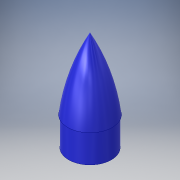
# Autodesk Inventor part: NoseCone
Saved by Autodesk Inventor 2018 (Build 220112000, 112)
## iProperties
Created: 2017-10-02
Part Number: NoseCone
Material: Generic
Document SubType Name: Modeling
Designer: Intel
Density: 1 g/cm^3
Appearance: Blue - Wall Paint - Glossy
Author: Intel
Autodesk Inventor part; units mm, degrees
ref_plane "YZ Plane" through (0, 0, 0) normal (1, 0, 0) x (0, 1, 0)
ref_plane "XZ Plane" through (0, 0, 0) normal (0, 1, 0) x (-1, 0, 0)
ref_plane "XY Plane" through (0, 0, 0) normal (0, 0, 1) x (1, 0, 0)
sketch "Sketch1" plane through (0, 0, 0) normal (0, 0, 1) x (1, 0, 0)
  line L0 (0, 0) -> (-39.6875, 0)
  line L1 (0, 0) -> (0, 127)
  arc A0 (0, 127) -> (-39.6875, 0) centre (313.5764, -40.6938) ccw
  line L2 (0, 0) -> (-38.1, 0)
  line L3 (-38.1, 0) -> (-38.1, -50.8)
  line L4 (-38.1, -50.8) -> (0, -50.8)
  line L5 (0, -50.8) -> (0, 0)
  dimension "d0" = 39.6875
  dimension "d1" = 127
  dimension "d3" = 355.6
  dimension "d5" = 38.1
  dimension "d6" = 50.8
  constraints: 12 end point, 2 horizontal, 2 parallel, 2 point on circle, 1 centre point, 1 perpendicular, 1 vertical
  measures "d0" distance of L0.start L0.end
  measures "d1" distance of L0.start L1.end
  measures "d3" radius of A0
  measures "d5" distance of L4.end L3.end
  measures "d6" distance between parallel lines of L0 L4
revolve "Revolution1" add sketch "Sketch1" angle 360 about axis through (0, 0, 0) along (0, 1, 0)
body "Solid1"
